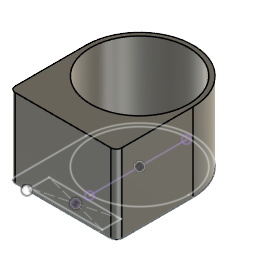
Refrigerator Marker Holder (Autodesk Fusion 360 design; units mm, degrees)
Autodesk Fusion 360 part; units mm, degrees
sketch "Sketch1" plane through (0, 0, 0) normal (0, 0, 1) x (1, 0, 0)
  line L0 (6.5, -1.7) -> (-6.5, -1.7)
  line L1 (-6.5, -1.7) -> (-6.5, 1.7)
  line L2 (-6.5, 1.7) -> (6.5, 1.7)
  line L3 (6.5, 1.7) -> (6.5, -1.7)
  line L4 (6.5, -1.7) -> (-6.5, 1.7) construction
  line L5 (-6.5, -1.7) -> (6.5, 1.7) construction
  line L6 (6.5, -2.3) -> (-6.5, -2.3)
  line L7 (6.5, -2.3) -> (9.65, -2.3)
  circle A0 centre (0, 11.55) radius 8.85
  line L8 (9.65, -2.3) -> (9.65, 11.55)
  line L9 (0, 2.5) -> (0, 20)
  line L10 (-6.5, -2.3) -> (-9.65, -2.3)
  line L11 (-9.65, -2.3) -> (-9.65, 11.55)
  arc A1 (9.65, 11.55) -> (-9.65, 11.55) centre (0, 11.55) ccw
  dimension "d1" = 13
  dimension "d2" = 3.4
  dimension "d3" = -0.6
  dimension "d4" = 17.7
  dimension "d5" = 1
  dimension "d6" = 0.8
  constraint horizontal L0
  constraint perpendicular L0 L1
  constraint parallel L0 L2
  constraint parallel L1 L3
  constraint coincident L4 origin
  constraint coincident L5 origin
  constraint parallel L6 L7
  constraint perpendicular L7 L8
  constraint horizontal A0.centre L8.end
  constraint symmetric L6.start L9 L6.end
  constraint symmetric L7.end L9 L10.end
  constraint symmetric L8.end L9 L11.end
  constraint coincident A0.centre A1.centre
  constraint coincident L11.end A1.end
  measures "d1" distance of L0.start L0.end
  measures "d2" distance of L0.end L1.end
  measures "d4" diameter of A0
  measures "d5" distance of L2 A0
  measures "d6" distance of A0 A1
extrude "Extrude1" add sketch "Sketch1" along normal blind 0.4 contours L0 L1 L2 L3 | L6 L7 L8 L10 L11 A1
extrude "Extrude2" add sketch "Sketch1" along normal blind 13 from surface at 0.4
extrude "Extrude3" add sketch "Sketch1" along normal blind 0.8 from surface at 13.4 contours L0 L1 L2 L3 | L6 L7 L8 L10 L11 A1
fillet "Fillet1" radius 1 2 edges at (9.65, -2.3, 7.1) (-9.65, -2.3, 7.1)
